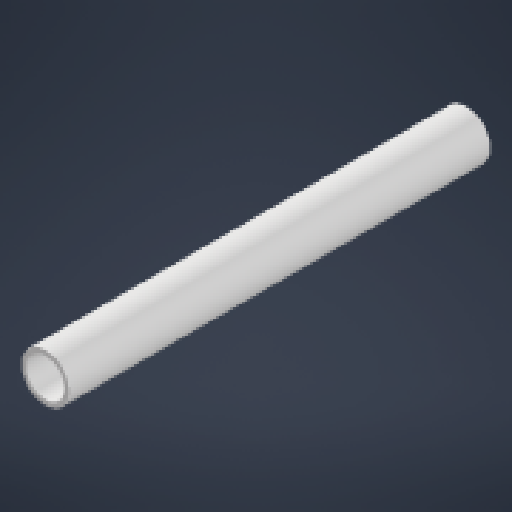
# Autodesk Inventor part: ClimberAxel
Saved by Autodesk Inventor 2024.3 (Build 283343000, 343)
## iProperties
Created: 2025-03-19
Part Number: ClimberAxel
Material: Aluminum 6061
Document SubType Name: Modeling
Designer: jings
Density: 2.7 g/cm^3
Appearance: Aluminum - Flat
Mass: 254.109 g
Surface Area: 598.548 cm^2
Volume: 94.1146 cm^3
Author: jings
Autodesk Inventor part; units mm, degrees
ref_plane "YZ Plane" through (0, 0, 0) normal (1, 0, 0) x (0, 1, 0)
ref_plane "XZ Plane" through (0, 0, 0) normal (0, 1, 0) x (-1, 0, 0)
ref_plane "XY Plane" through (0, 0, 0) normal (0, 0, 1) x (1, 0, 0)
sketch "Sketch1" plane through (0, 0, 0) normal (0, 0, 1) x (1, 0, 0)
  circle A0 centre (0, 0) radius 12.7
  circle A1 centre (0, 0) radius 15.875
  dimension "d2" = 31.75
  dimension "d5" = 3.175
  constraints: 2 centre point, 2 coincident
  measures "d2" diameter of A1
  measures "d5" radial gap between concentric circles of A1 A0
extrude "Extrusion1" add sketch "Sketch1" along normal mid plane 330.2
body "Solid1"
